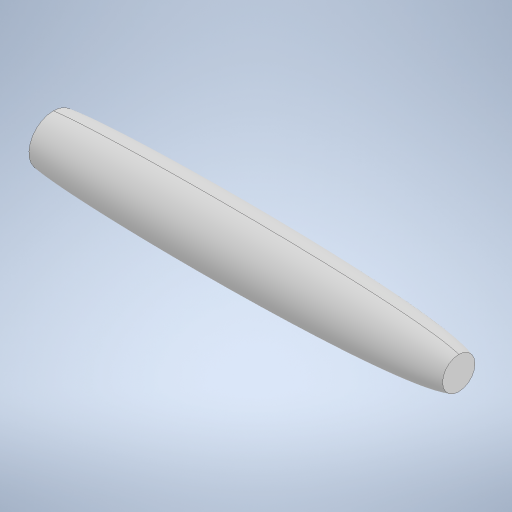
# Autodesk Inventor part: Part1.iptarker
Saved by Autodesk Inventor 2023 (Build 270158030, 158C)
## iProperties
Created: 2024-03-10
Part Number: Part1.iptarker
Material: Generic
Document SubType Name: Modeling
Designer: Imogen Heard
Density: 1 g/cm^3
Appearance: Default
Author: Imogen Heard
Autodesk Inventor part; units mm, degrees
ref_plane "YZ Plane" through (0, 0, 0) normal (1, 0, 0) x (0, 1, 0)
ref_plane "XZ Plane" through (0, 0, 0) normal (0, 1, 0) x (-1, 0, 0)
ref_plane "XY Plane" through (0, 0, 0) normal (0, 0, 1) x (1, 0, 0)
sketch "Sketch3" plane through (0, 0, 0) normal (0, 0, 1) x (1, 0, 0)
  line L0 (50, 4) -> (50, 0)
  line L1 (50, 0) -> (-50, 0)
  line L2 (-50, 0) -> (-50, 6)
  line L3 (-50, 6) -> (-43, 7) construction
  line L4 (-43, 7) -> (-20, 8) construction
  line L5 (-20, 8) -> (38, 8) construction
  line L6 (38, 8) -> (50, 4) construction
  spline S0 degree 4 poles (-50, 6) (-43, 7) (-20, 8) (38, 8) (50, 4) knots 1 1 1 1 1 2 2 2 2 2
  point P0 (0, 0)
  dimension "d1" = 100
  dimension "d2" = 6
  dimension "d3" = 4
  dimension "d4" = 7
  dimension "d5" = 8
  dimension "d6" = 8
  dimension "d7" = 38
  dimension "d8" = 20
  dimension "d9" = 43
  dimension "d10" = 50
  constraints: 6 end point, 1 horizontal alignment, 1 parallel, 3 other
  measures "d1" distance between parallel lines of L0 L2
  measures "d2" vertical distance of L2.end point (0, 0)
  measures "d3" vertical distance of point (0, 0) L0.start
  measures "d4" vertical distance of point (0, 0) L3.end
  measures "d5" vertical distance of point (0, 0) L4.end
  measures "d6" vertical distance of point (0, 0) L5.end
  measures "d7" horizontal distance of point (0, 0) L5.end
  measures "d8" horizontal distance of L4.end point (0, 0)
  measures "d9" horizontal distance of point (0, 0) L3.end
  measures "d10" distance of point (0, 0) L1.end
revolve "Revolution1" add sketch "Sketch3" angle 360 about axis through (50, 0, 0) along (-1, 0, 0)
equation "\"d10\" = 0.5 * d1"
body "Solid1"
